Autodesk Inventor part; units mm, degrees
(part 4 of 5)
  line L871 (-97.2926, -57.6618) -> (-97.2926, -57.0118) projected
  line L872 (-97.2926, -49.1118) -> (-95.6926, -49.1118) projected
  line L873 (-95.6926, -49.1118) -> (-95.6926, -49.7618) projected
  line L874 (-95.6926, -49.7618) -> (-97.2926, -49.7618) projected
  line L875 (-97.2926, -49.7618) -> (-97.2926, -49.1118) projected
  line L876 (-98.1576, -55.9868) -> (-97.3676, -55.9868) projected
  line L877 (-97.3676, -55.9868) -> (-97.3676, -56.3868) projected
  line L878 (-97.3676, -56.3868) -> (-98.1576, -56.3868) projected
  line L879 (-98.1576, -56.3868) -> (-98.1576, -55.9868) projected
  line L880 (-95.6176, -55.9868) -> (-94.8276, -55.9868) projected
  line L881 (-94.8276, -55.9868) -> (-94.8276, -56.3868) projected
  line L882 (-94.8276, -56.3868) -> (-95.6176, -56.3868) projected
  line L883 (-95.6176, -56.3868) -> (-95.6176, -55.9868) projected
  line L884 (-98.1576, -55.1868) -> (-97.3676, -55.1868) projected
  line L885 (-97.3676, -55.1868) -> (-97.3676, -55.5868) projected
  line L886 (-97.3676, -55.5868) -> (-98.1576, -55.5868) projected
  line L887 (-98.1576, -55.5868) -> (-98.1576, -55.1868) projected
  line L888 (-95.6176, -55.1868) -> (-94.8276, -55.1868) projected
  line L889 (-94.8276, -55.1868) -> (-94.8276, -55.5868) projected
  line L890 (-94.8276, -55.5868) -> (-95.6176, -55.5868) projected
  line L891 (-95.6176, -55.5868) -> (-95.6176, -55.1868) projected
  line L892 (-98.1576, -54.3868) -> (-97.3676, -54.3868) projected
  line L893 (-97.3676, -54.3868) -> (-97.3676, -54.7868) projected
  line L894 (-97.3676, -54.7868) -> (-98.1576, -54.7868) projected
  line L895 (-98.1576, -54.7868) -> (-98.1576, -54.3868) projected
  line L896 (-95.6176, -54.3868) -> (-94.8276, -54.3868) projected
  line L897 (-94.8276, -54.3868) -> (-94.8276, -54.7868) projected
  line L898 (-94.8276, -54.7868) -> (-95.6176, -54.7868) projected
  line L899 (-95.6176, -54.7868) -> (-95.6176, -54.3868) projected
  line L900 (-98.1576, -53.5868) -> (-97.3676, -53.5868) projected
  line L901 (-97.3676, -53.5868) -> (-97.3676, -53.9868) projected
  line L902 (-97.3676, -53.9868) -> (-98.1576, -53.9868) projected
  line L903 (-98.1576, -53.9868) -> (-98.1576, -53.5868) projected
  line L904 (-95.6176, -53.5868) -> (-94.8276, -53.5868) projected
  line L905 (-94.8276, -53.5868) -> (-94.8276, -53.9868) projected
  line L906 (-94.8276, -53.9868) -> (-95.6176, -53.9868) projected
  line L907 (-95.6176, -53.9868) -> (-95.6176, -53.5868) projected
  line L908 (-98.1576, -52.7868) -> (-97.3676, -52.7868) projected
  line L909 (-97.3676, -52.7868) -> (-97.3676, -53.1868) projected
  line L910 (-97.3676, -53.1868) -> (-98.1576, -53.1868) projected
  line L911 (-98.1576, -53.1868) -> (-98.1576, -52.7868) projected
  line L912 (-95.6176, -52.7868) -> (-94.8276, -52.7868) projected
  line L913 (-94.8276, -52.7868) -> (-94.8276, -53.1868) projected
  line L914 (-94.8276, -53.1868) -> (-95.6176, -53.1868) projected
  line L915 (-95.6176, -53.1868) -> (-95.6176, -52.7868) projected
  line L916 (-98.1576, -51.9868) -> (-97.3676, -51.9868) projected
  line L917 (-97.3676, -51.9868) -> (-97.3676, -52.3868) projected
  line L918 (-97.3676, -52.3868) -> (-98.1576, -52.3868) projected
  line L919 (-98.1576, -52.3868) -> (-98.1576, -51.9868) projected
  line L920 (-95.6176, -51.9868) -> (-94.8276, -51.9868) projected
  line L921 (-94.8276, -51.9868) -> (-94.8276, -52.3868) projected
  line L922 (-94.8276, -52.3868) -> (-95.6176, -52.3868) projected
  line L923 (-95.6176, -52.3868) -> (-95.6176, -51.9868) projected
  line L924 (-98.1576, -51.1868) -> (-97.3676, -51.1868) projected
  line L925 (-97.3676, -51.1868) -> (-97.3676, -51.5868) projected
  line L926 (-97.3676, -51.5868) -> (-98.1576, -51.5868) projected
  line L927 (-98.1576, -51.5868) -> (-98.1576, -51.1868) projected
  line L928 (-95.6176, -51.1868) -> (-94.8276, -51.1868) projected
  line L929 (-94.8276, -51.1868) -> (-94.8276, -51.5868) projected
  line L930 (-94.8276, -51.5868) -> (-95.6176, -51.5868) projected
  line L931 (-95.6176, -51.5868) -> (-95.6176, -51.1868) projected
  line L932 (-98.1576, -50.3868) -> (-97.3676, -50.3868) projected
  line L933 (-97.3676, -50.3868) -> (-97.3676, -50.7868) projected
  line L934 (-97.3676, -50.7868) -> (-98.1576, -50.7868) projected
  line L935 (-98.1576, -50.7868) -> (-98.1576, -50.3868) projected
  line L936 (-95.6176, -50.3868) -> (-94.8276, -50.3868) projected
  line L937 (-94.8276, -50.3868) -> (-94.8276, -50.7868) projected
  line L938 (-94.8276, -50.7868) -> (-95.6176, -50.7868) projected
  line L939 (-95.6176, -50.7868) -> (-95.6176, -50.3868) projected
  line L940 (-59.7501, -19.4368) -> (-58.1501, -19.4368) projected
  line L941 (-58.1501, -19.4368) -> (-58.1501, -20.0868) projected
  line L942 (-58.1501, -20.0868) -> (-59.7501, -20.0868) projected
  line L943 (-59.7501, -20.0868) -> (-59.7501, -19.4368) projected
  line L944 (-59.7501, -11.5368) -> (-58.1501, -11.5368) projected
  line L945 (-58.1501, -11.5368) -> (-58.1501, -12.1868) projected
  line L946 (-58.1501, -12.1868) -> (-59.7501, -12.1868) projected
  line L947 (-59.7501, -12.1868) -> (-59.7501, -11.5368) projected
  line L948 (-60.6151, -18.4118) -> (-59.8251, -18.4118) projected
  line L949 (-59.8251, -18.4118) -> (-59.8251, -18.8118) projected
  line L950 (-59.8251, -18.8118) -> (-60.6151, -18.8118) projected
  line L951 (-60.6151, -18.8118) -> (-60.6151, -18.4118) projected
  line L952 (-58.0751, -18.4118) -> (-57.2851, -18.4118) projected
  line L953 (-57.2851, -18.4118) -> (-57.2851, -18.8118) projected
  line L954 (-57.2851, -18.8118) -> (-58.0751, -18.8118) projected
  line L955 (-58.0751, -18.8118) -> (-58.0751, -18.4118) projected
  line L956 (-60.6151, -17.6118) -> (-59.8251, -17.6118) projected
  line L957 (-59.8251, -17.6118) -> (-59.8251, -18.0118) projected
  line L958 (-59.8251, -18.0118) -> (-60.6151, -18.0118) projected
  line L959 (-60.6151, -18.0118) -> (-60.6151, -17.6118) projected
  line L960 (-58.0751, -17.6118) -> (-57.2851, -17.6118) projected
  line L961 (-57.2851, -17.6118) -> (-57.2851, -18.0118) projected
  line L962 (-57.2851, -18.0118) -> (-58.0751, -18.0118) projected
  line L963 (-58.0751, -18.0118) -> (-58.0751, -17.6118) projected
  line L964 (-60.6151, -16.8118) -> (-59.8251, -16.8118) projected
  line L965 (-59.8251, -16.8118) -> (-59.8251, -17.2118) projected
  line L966 (-59.8251, -17.2118) -> (-60.6151, -17.2118) projected
  line L967 (-60.6151, -17.2118) -> (-60.6151, -16.8118) projected
  line L968 (-58.0751, -16.8118) -> (-57.2851, -16.8118) projected
  line L969 (-57.2851, -16.8118) -> (-57.2851, -17.2118) projected
  line L970 (-57.2851, -17.2118) -> (-58.0751, -17.2118) projected
  line L971 (-58.0751, -17.2118) -> (-58.0751, -16.8118) projected
  line L972 (-60.6151, -16.0118) -> (-59.8251, -16.0118) projected
  line L973 (-59.8251, -16.0118) -> (-59.8251, -16.4118) projected
  line L974 (-59.8251, -16.4118) -> (-60.6151, -16.4118) projected
  line L975 (-60.6151, -16.4118) -> (-60.6151, -16.0118) projected
  line L976 (-58.0751, -16.0118) -> (-57.2851, -16.0118) projected
  line L977 (-57.2851, -16.0118) -> (-57.2851, -16.4118) projected
  line L978 (-57.2851, -16.4118) -> (-58.0751, -16.4118) projected
  line L979 (-58.0751, -16.4118) -> (-58.0751, -16.0118) projected
  line L980 (-60.6151, -15.2118) -> (-59.8251, -15.2118) projected
  line L981 (-59.8251, -15.2118) -> (-59.8251, -15.6118) projected
  line L982 (-59.8251, -15.6118) -> (-60.6151, -15.6118) projected
  line L983 (-60.6151, -15.6118) -> (-60.6151, -15.2118) projected
  line L984 (-58.0751, -15.2118) -> (-57.2851, -15.2118) projected
  line L985 (-57.2851, -15.2118) -> (-57.2851, -15.6118) projected
  line L986 (-57.2851, -15.6118) -> (-58.0751, -15.6118) projected
  line L987 (-58.0751, -15.6118) -> (-58.0751, -15.2118) projected
  line L988 (-60.6151, -14.4118) -> (-59.8251, -14.4118) projected
  line L989 (-59.8251, -14.4118) -> (-59.8251, -14.8118) projected
  line L990 (-59.8251, -14.8118) -> (-60.6151, -14.8118) projected
  line L991 (-60.6151, -14.8118) -> (-60.6151, -14.4118) projected
  line L992 (-58.0751, -14.4118) -> (-57.2851, -14.4118) projected
  line L993 (-57.2851, -14.4118) -> (-57.2851, -14.8118) projected
  line L994 (-57.2851, -14.8118) -> (-58.0751, -14.8118) projected
  line L995 (-58.0751, -14.8118) -> (-58.0751, -14.4118) projected
  line L996 (-60.6151, -13.6118) -> (-59.8251, -13.6118) projected
  line L997 (-59.8251, -13.6118) -> (-59.8251, -14.0118) projected
  line L998 (-59.8251, -14.0118) -> (-60.6151, -14.0118) projected
  line L999 (-60.6151, -14.0118) -> (-60.6151, -13.6118) projected
  line L1000 (-58.0751, -13.6118) -> (-57.2851, -13.6118) projected
  line L1001 (-57.2851, -13.6118) -> (-57.2851, -14.0118) projected
  line L1002 (-57.2851, -14.0118) -> (-58.0751, -14.0118) projected
  line L1003 (-58.0751, -14.0118) -> (-58.0751, -13.6118) projected
  line L1004 (-60.6151, -12.8118) -> (-59.8251, -12.8118) projected
  line L1005 (-59.8251, -12.8118) -> (-59.8251, -13.2118) projected
  line L1006 (-59.8251, -13.2118) -> (-60.6151, -13.2118) projected
  line L1007 (-60.6151, -13.2118) -> (-60.6151, -12.8118) projected
  line L1008 (-58.0751, -12.8118) -> (-57.2851, -12.8118) projected
  line L1009 (-57.2851, -12.8118) -> (-57.2851, -13.2118) projected
  line L1010 (-57.2851, -13.2118) -> (-58.0751, -13.2118) projected
  line L1011 (-58.0751, -13.2118) -> (-58.0751, -12.8118) projected
  line L1012 (-116.5001, -19.3118) -> (-114.9001, -19.3118) projected
  line L1013 (-114.9001, -19.3118) -> (-114.9001, -19.9618) projected
  line L1014 (-114.9001, -19.9618) -> (-116.5001, -19.9618) projected
  line L1015 (-116.5001, -19.9618) -> (-116.5001, -19.3118) projected
  line L1016 (-116.5001, -11.4118) -> (-114.9001, -11.4118) projected
  line L1017 (-114.9001, -11.4118) -> (-114.9001, -12.0618) projected
  line L1018 (-114.9001, -12.0618) -> (-116.5001, -12.0618) projected
  line L1019 (-116.5001, -12.0618) -> (-116.5001, -11.4118) projected
  line L1020 (-117.3651, -18.2868) -> (-116.5751, -18.2868) projected
  line L1021 (-116.5751, -18.2868) -> (-116.5751, -18.6868) projected
  line L1022 (-116.5751, -18.6868) -> (-117.3651, -18.6868) projected
  line L1023 (-117.3651, -18.6868) -> (-117.3651, -18.2868) projected
  line L1024 (-114.8251, -18.2868) -> (-114.0351, -18.2868) projected
  line L1025 (-114.0351, -18.2868) -> (-114.0351, -18.6868) projected
  line L1026 (-114.0351, -18.6868) -> (-114.8251, -18.6868) projected
  line L1027 (-114.8251, -18.6868) -> (-114.8251, -18.2868) projected
  line L1028 (-117.3651, -17.4868) -> (-116.5751, -17.4868) projected
  line L1029 (-116.5751, -17.4868) -> (-116.5751, -17.8868) projected
  line L1030 (-116.5751, -17.8868) -> (-117.3651, -17.8868) projected
  line L1031 (-117.3651, -17.8868) -> (-117.3651, -17.4868) projected
  line L1032 (-114.8251, -17.4868) -> (-114.0351, -17.4868) projected
  line L1033 (-114.0351, -17.4868) -> (-114.0351, -17.8868) projected
  line L1034 (-114.0351, -17.8868) -> (-114.8251, -17.8868) projected
  line L1035 (-114.8251, -17.8868) -> (-114.8251, -17.4868) projected
  line L1036 (-117.3651, -16.6868) -> (-116.5751, -16.6868) projected
  line L1037 (-116.5751, -16.6868) -> (-116.5751, -17.0868) projected
  line L1038 (-116.5751, -17.0868) -> (-117.3651, -17.0868) projected
  line L1039 (-117.3651, -17.0868) -> (-117.3651, -16.6868) projected
  line L1040 (-114.8251, -16.6868) -> (-114.0351, -16.6868) projected
  line L1041 (-114.0351, -16.6868) -> (-114.0351, -17.0868) projected
  line L1042 (-114.0351, -17.0868) -> (-114.8251, -17.0868) projected
  line L1043 (-114.8251, -17.0868) -> (-114.8251, -16.6868) projected
  line L1044 (-117.3651, -15.8868) -> (-116.5751, -15.8868) projected
  line L1045 (-116.5751, -15.8868) -> (-116.5751, -16.2868) projected
  line L1046 (-116.5751, -16.2868) -> (-117.3651, -16.2868) projected
  line L1047 (-117.3651, -16.2868) -> (-117.3651, -15.8868) projected
  line L1048 (-114.8251, -15.8868) -> (-114.0351, -15.8868) projected
  line L1049 (-114.0351, -15.8868) -> (-114.0351, -16.2868) projected
  line L1050 (-114.0351, -16.2868) -> (-114.8251, -16.2868) projected
  line L1051 (-114.8251, -16.2868) -> (-114.8251, -15.8868) projected
  line L1052 (-117.3651, -15.0868) -> (-116.5751, -15.0868) projected
  line L1053 (-116.5751, -15.0868) -> (-116.5751, -15.4868) projected
  line L1054 (-116.5751, -15.4868) -> (-117.3651, -15.4868) projected
  line L1055 (-117.3651, -15.4868) -> (-117.3651, -15.0868) projected
  line L1056 (-114.8251, -15.0868) -> (-114.0351, -15.0868) projected
  line L1057 (-114.0351, -15.0868) -> (-114.0351, -15.4868) projected
  line L1058 (-114.0351, -15.4868) -> (-114.8251, -15.4868) projected
  line L1059 (-114.8251, -15.4868) -> (-114.8251, -15.0868) projected
  line L1060 (-117.3651, -14.2868) -> (-116.5751, -14.2868) projected
  line L1061 (-116.5751, -14.2868) -> (-116.5751, -14.6868) projected
  line L1062 (-116.5751, -14.6868) -> (-117.3651, -14.6868) projected
  line L1063 (-117.3651, -14.6868) -> (-117.3651, -14.2868) projected
  line L1064 (-114.8251, -14.2868) -> (-114.0351, -14.2868) projected
  line L1065 (-114.0351, -14.2868) -> (-114.0351, -14.6868) projected
  line L1066 (-114.0351, -14.6868) -> (-114.8251, -14.6868) projected
  line L1067 (-114.8251, -14.6868) -> (-114.8251, -14.2868) projected
  line L1068 (-117.3651, -13.4868) -> (-116.5751, -13.4868) projected
  line L1069 (-116.5751, -13.4868) -> (-116.5751, -13.8868) projected
  line L1070 (-116.5751, -13.8868) -> (-117.3651, -13.8868) projected
  line L1071 (-117.3651, -13.8868) -> (-117.3651, -13.4868) projected
  line L1072 (-114.8251, -13.4868) -> (-114.0351, -13.4868) projected
  line L1073 (-114.0351, -13.4868) -> (-114.0351, -13.8868) projected
  line L1074 (-114.0351, -13.8868) -> (-114.8251, -13.8868) projected
  line L1075 (-114.8251, -13.8868) -> (-114.8251, -13.4868) projected
  line L1076 (-117.3651, -12.6868) -> (-116.5751, -12.6868) projected
  line L1077 (-116.5751, -12.6868) -> (-116.5751, -13.0868) projected
  line L1078 (-116.5751, -13.0868) -> (-117.3651, -13.0868) projected
  line L1079 (-117.3651, -13.0868) -> (-117.3651, -12.6868) projected
  line L1080 (-114.8251, -12.6868) -> (-114.0351, -12.6868) projected
  line L1081 (-114.0351, -12.6868) -> (-114.0351, -13.0868) projected
  line L1082 (-114.0351, -13.0868) -> (-114.8251, -13.0868) projected
  line L1083 (-114.8251, -13.0868) -> (-114.8251, -12.6868) projected
  line L1084 (-40.9426, -19.3618) -> (-39.3426, -19.3618) projected
  line L1085 (-39.3426, -19.3618) -> (-39.3426, -20.0118) projected
  line L1086 (-39.3426, -20.0118) -> (-40.9426, -20.0118) projected
  line L1087 (-40.9426, -20.0118) -> (-40.9426, -19.3618) projected
  line L1088 (-40.9426, -11.4618) -> (-39.3426, -11.4618) projected
  line L1089 (-39.3426, -11.4618) -> (-39.3426, -12.1118) projected
  line L1090 (-39.3426, -12.1118) -> (-40.9426, -12.1118) projected
  line L1091 (-40.9426, -12.1118) -> (-40.9426, -11.4618) projected
  line L1092 (-41.8076, -18.3368) -> (-41.0176, -18.3368) projected
  line L1093 (-41.0176, -18.3368) -> (-41.0176, -18.7368) projected
  line L1094 (-41.0176, -18.7368) -> (-41.8076, -18.7368) projected
  line L1095 (-41.8076, -18.7368) -> (-41.8076, -18.3368) projected
  line L1096 (-39.2676, -18.3368) -> (-38.4776, -18.3368) projected
  line L1097 (-38.4776, -18.3368) -> (-38.4776, -18.7368) projected
  line L1098 (-38.4776, -18.7368) -> (-39.2676, -18.7368) projected
  line L1099 (-39.2676, -18.7368) -> (-39.2676, -18.3368) projected
  line L1100 (-41.8076, -17.5368) -> (-41.0176, -17.5368) projected
  line L1101 (-41.0176, -17.5368) -> (-41.0176, -17.9368) projected
  line L1102 (-41.0176, -17.9368) -> (-41.8076, -17.9368) projected
  line L1103 (-41.8076, -17.9368) -> (-41.8076, -17.5368) projected
  line L1104 (-39.2676, -17.5368) -> (-38.4776, -17.5368) projected
  line L1105 (-38.4776, -17.5368) -> (-38.4776, -17.9368) projected
  line L1106 (-38.4776, -17.9368) -> (-39.2676, -17.9368) projected
  line L1107 (-39.2676, -17.9368) -> (-39.2676, -17.5368) projected
  line L1108 (-41.8076, -16.7368) -> (-41.0176, -16.7368) projected
  line L1109 (-41.0176, -16.7368) -> (-41.0176, -17.1368) projected
  line L1110 (-41.0176, -17.1368) -> (-41.8076, -17.1368) projected
  line L1111 (-41.8076, -17.1368) -> (-41.8076, -16.7368) projected
  line L1112 (-39.2676, -16.7368) -> (-38.4776, -16.7368) projected
  line L1113 (-38.4776, -16.7368) -> (-38.4776, -17.1368) projected
  line L1114 (-38.4776, -17.1368) -> (-39.2676, -17.1368) projected
  line L1115 (-39.2676, -17.1368) -> (-39.2676, -16.7368) projected
  line L1116 (-41.8076, -15.9368) -> (-41.0176, -15.9368) projected
  line L1117 (-41.0176, -15.9368) -> (-41.0176, -16.3368) projected
  line L1118 (-41.0176, -16.3368) -> (-41.8076, -16.3368) projected
  line L1119 (-41.8076, -16.3368) -> (-41.8076, -15.9368) projected
  line L1120 (-39.2676, -15.9368) -> (-38.4776, -15.9368) projected
  line L1121 (-38.4776, -15.9368) -> (-38.4776, -16.3368) projected
  line L1122 (-38.4776, -16.3368) -> (-39.2676, -16.3368) projected
  line L1123 (-39.2676, -16.3368) -> (-39.2676, -15.9368) projected
  line L1124 (-41.8076, -15.1368) -> (-41.0176, -15.1368) projected
  line L1125 (-41.0176, -15.1368) -> (-41.0176, -15.5368) projected
  line L1126 (-41.0176, -15.5368) -> (-41.8076, -15.5368) projected
  line L1127 (-41.8076, -15.5368) -> (-41.8076, -15.1368) projected
  line L1128 (-39.2676, -15.1368) -> (-38.4776, -15.1368) projected
  line L1129 (-38.4776, -15.1368) -> (-38.4776, -15.5368) projected
  line L1130 (-38.4776, -15.5368) -> (-39.2676, -15.5368) projected
  line L1131 (-39.2676, -15.5368) -> (-39.2676, -15.1368) projected
  line L1132 (-41.8076, -14.3368) -> (-41.0176, -14.3368) projected
  line L1133 (-41.0176, -14.3368) -> (-41.0176, -14.7368) projected
  line L1134 (-41.0176, -14.7368) -> (-41.8076, -14.7368) projected
  line L1135 (-41.8076, -14.7368) -> (-41.8076, -14.3368) projected
  line L1136 (-39.2676, -14.3368) -> (-38.4776, -14.3368) projected
  line L1137 (-38.4776, -14.3368) -> (-38.4776, -14.7368) projected
  line L1138 (-38.4776, -14.7368) -> (-39.2676, -14.7368) projected
  line L1139 (-39.2676, -14.7368) -> (-39.2676, -14.3368) projected
  line L1140 (-41.8076, -13.5368) -> (-41.0176, -13.5368) projected
  line L1141 (-41.0176, -13.5368) -> (-41.0176, -13.9368) projected
  line L1142 (-41.0176, -13.9368) -> (-41.8076, -13.9368) projected
  line L1143 (-41.8076, -13.9368) -> (-41.8076, -13.5368) projected
  line L1144 (-39.2676, -13.5368) -> (-38.4776, -13.5368) projected
  line L1145 (-38.4776, -13.5368) -> (-38.4776, -13.9368) projected
  line L1146 (-38.4776, -13.9368) -> (-39.2676, -13.9368) projected
  line L1147 (-39.2676, -13.9368) -> (-39.2676, -13.5368) projected
  line L1148 (-41.8076, -12.7368) -> (-41.0176, -12.7368) projected
  line L1149 (-41.0176, -12.7368) -> (-41.0176, -13.1368) projected
  line L1150 (-41.0176, -13.1368) -> (-41.8076, -13.1368) projected
  line L1151 (-41.8076, -13.1368) -> (-41.8076, -12.7368) projected
  line L1152 (-39.2676, -12.7368) -> (-38.4776, -12.7368) projected
  line L1153 (-38.4776, -12.7368) -> (-38.4776, -13.1368) projected
  line L1154 (-38.4776, -13.1368) -> (-39.2676, -13.1368) projected
  line L1155 (-39.2676, -13.1368) -> (-39.2676, -12.7368) projected
  line L1156 (-40.7851, -57.0368) -> (-39.1851, -57.0368) projected
  line L1157 (-39.1851, -57.0368) -> (-39.1851, -57.6868) projected
  line L1158 (-39.1851, -57.6868) -> (-40.7851, -57.6868) projected
  line L1159 (-40.7851, -57.6868) -> (-40.7851, -57.0368) projected
  line L1160 (-40.7851, -49.1368) -> (-39.1851, -49.1368) projected
  line L1161 (-39.1851, -49.1368) -> (-39.1851, -49.7868) projected
  line L1162 (-39.1851, -49.7868) -> (-40.7851, -49.7868) projected
  line L1163 (-40.7851, -49.7868) -> (-40.7851, -49.1368) projected
  line L1164 (-41.6501, -56.0118) -> (-40.8601, -56.0118) projected
  line L1165 (-40.8601, -56.0118) -> (-40.8601, -56.4118) projected
  line L1166 (-40.8601, -56.4118) -> (-41.6501, -56.4118) projected
  line L1167 (-41.6501, -56.4118) -> (-41.6501, -56.0118) projected
  line L1168 (-39.1101, -56.0118) -> (-38.3201, -56.0118) projected
  line L1169 (-38.3201, -56.0118) -> (-38.3201, -56.4118) projected
  line L1170 (-38.3201, -56.4118) -> (-39.1101, -56.4118) projected
  line L1171 (-39.1101, -56.4118) -> (-39.1101, -56.0118) projected
  line L1172 (-41.6501, -55.2118) -> (-40.8601, -55.2118) projected
  line L1173 (-40.8601, -55.2118) -> (-40.8601, -55.6118) projected
  line L1174 (-40.8601, -55.6118) -> (-41.6501, -55.6118) projected
  line L1175 (-41.6501, -55.6118) -> (-41.6501, -55.2118) projected
  line L1176 (-39.1101, -55.2118) -> (-38.3201, -55.2118) projected
  line L1177 (-38.3201, -55.2118) -> (-38.3201, -55.6118) projected
  line L1178 (-38.3201, -55.6118) -> (-39.1101, -55.6118) projected
  line L1179 (-39.1101, -55.6118) -> (-39.1101, -55.2118) projected
  line L1180 (-41.6501, -54.4118) -> (-40.8601, -54.4118) projected
  line L1181 (-40.8601, -54.4118) -> (-40.8601, -54.8118) projected
  line L1182 (-40.8601, -54.8118) -> (-41.6501, -54.8118) projected
  line L1183 (-41.6501, -54.8118) -> (-41.6501, -54.4118) projected
  line L1184 (-39.1101, -54.4118) -> (-38.3201, -54.4118) projected
  line L1185 (-38.3201, -54.4118) -> (-38.3201, -54.8118) projected
  line L1186 (-38.3201, -54.8118) -> (-39.1101, -54.8118) projected
  line L1187 (-39.1101, -54.8118) -> (-39.1101, -54.4118) projected
  line L1188 (-41.6501, -53.6118) -> (-40.8601, -53.6118) projected
  line L1189 (-40.8601, -53.6118) -> (-40.8601, -54.0118) projected
  line L1190 (-40.8601, -54.0118) -> (-41.6501, -54.0118) projected
  line L1191 (-41.6501, -54.0118) -> (-41.6501, -53.6118) projected
  line L1192 (-39.1101, -53.6118) -> (-38.3201, -53.6118) projected
  line L1193 (-38.3201, -53.6118) -> (-38.3201, -54.0118) projected
  line L1194 (-38.3201, -54.0118) -> (-39.1101, -54.0118) projected
  line L1195 (-39.1101, -54.0118) -> (-39.1101, -53.6118) projected
  line L1196 (-41.6501, -52.8118) -> (-40.8601, -52.8118) projected
  line L1197 (-40.8601, -52.8118) -> (-40.8601, -53.2118) projected
  line L1198 (-40.8601, -53.2118) -> (-41.6501, -53.2118) projected
  line L1199 (-41.6501, -53.2118) -> (-41.6501, -52.8118) projected
  line L1200 (-39.1101, -52.8118) -> (-38.3201, -52.8118) projected
  line L1201 (-38.3201, -52.8118) -> (-38.3201, -53.2118) projected
  line L1202 (-38.3201, -53.2118) -> (-39.1101, -53.2118) projected
  line L1203 (-39.1101, -53.2118) -> (-39.1101, -52.8118) projected
  line L1204 (-41.6501, -52.0118) -> (-40.8601, -52.0118) projected
  line L1205 (-40.8601, -52.0118) -> (-40.8601, -52.4118) projected
  line L1206 (-40.8601, -52.4118) -> (-41.6501, -52.4118) projected
  line L1207 (-41.6501, -52.4118) -> (-41.6501, -52.0118) projected
  line L1208 (-39.1101, -52.0118) -> (-38.3201, -52.0118) projected
  line L1209 (-38.3201, -52.0118) -> (-38.3201, -52.4118) projected
  line L1210 (-38.3201, -52.4118) -> (-39.1101, -52.4118) projected
  line L1211 (-39.1101, -52.4118) -> (-39.1101, -52.0118) projected
  line L1212 (-41.6501, -51.2118) -> (-40.8601, -51.2118) projected
  line L1213 (-40.8601, -51.2118) -> (-40.8601, -51.6118) projected
  line L1214 (-40.8601, -51.6118) -> (-41.6501, -51.6118) projected
  line L1215 (-41.6501, -51.6118) -> (-41.6501, -51.2118) projected
  line L1216 (-39.1101, -51.2118) -> (-38.3201, -51.2118) projected
  line L1217 (-38.3201, -51.2118) -> (-38.3201, -51.6118) projected
  line L1218 (-38.3201, -51.6118) -> (-39.1101, -51.6118) projected
  line L1219 (-39.1101, -51.6118) -> (-39.1101, -51.2118) projected
  line L1220 (-41.6501, -50.4118) -> (-40.8601, -50.4118) projected
  line L1221 (-40.8601, -50.4118) -> (-40.8601, -50.8118) projected
  line L1222 (-40.8601, -50.8118) -> (-41.6501, -50.8118) projected
  line L1223 (-41.6501, -50.8118) -> (-41.6501, -50.4118) projected
  line L1224 (-39.1101, -50.4118) -> (-38.3201, -50.4118) projected
  line L1225 (-38.3201, -50.4118) -> (-38.3201, -50.8118) projected
  line L1226 (-38.3201, -50.8118) -> (-39.1101, -50.8118) projected
  line L1227 (-39.1101, -50.8118) -> (-39.1101, -50.4118) projected
  line L1228 (-78.4676, -57.1118) -> (-76.8676, -57.1118) projected
  line L1229 (-76.8676, -57.1118) -> (-76.8676, -57.7618) projected
  line L1230 (-76.8676, -57.7618) -> (-78.4676, -57.7618) projected
  line L1231 (-78.4676, -57.7618) -> (-78.4676, -57.1118) projected
  line L1232 (-78.4676, -49.2118) -> (-76.8676, -49.2118) projected
  line L1233 (-76.8676, -49.2118) -> (-76.8676, -49.8618) projected
  line L1234 (-76.8676, -49.8618) -> (-78.4676, -49.8618) projected
  line L1235 (-78.4676, -49.8618) -> (-78.4676, -49.2118) projected
  line L1236 (-79.3326, -56.0868) -> (-78.5426, -56.0868) projected
  line L1237 (-78.5426, -56.0868) -> (-78.5426, -56.4868) projected
  line L1238 (-78.5426, -56.4868) -> (-79.3326, -56.4868) projected
  line L1239 (-79.3326, -56.4868) -> (-79.3326, -56.0868) projected
  line L1240 (-76.7926, -56.0868) -> (-76.0026, -56.0868) projected
  line L1241 (-76.0026, -56.0868) -> (-76.0026, -56.4868) projected
  line L1242 (-76.0026, -56.4868) -> (-76.7926, -56.4868) projected
  line L1243 (-76.7926, -56.4868) -> (-76.7926, -56.0868) projected
  line L1244 (-79.3326, -55.2868) -> (-78.5426, -55.2868) projected
  line L1245 (-78.5426, -55.2868) -> (-78.5426, -55.6868) projected
  line L1246 (-78.5426, -55.6868) -> (-79.3326, -55.6868) projected
  line L1247 (-79.3326, -55.6868) -> (-79.3326, -55.2868) projected
  line L1248 (-76.7926, -55.2868) -> (-76.0026, -55.2868) projected
  line L1249 (-76.0026, -55.2868) -> (-76.0026, -55.6868) projected
  line L1250 (-76.0026, -55.6868) -> (-76.7926, -55.6868) projected
  line L1251 (-76.7926, -55.6868) -> (-76.7926, -55.2868) projected
  line L1252 (-79.3326, -54.4868) -> (-78.5426, -54.4868) projected
  line L1253 (-78.5426, -54.4868) -> (-78.5426, -54.8868) projected
  line L1254 (-78.5426, -54.8868) -> (-79.3326, -54.8868) projected
  line L1255 (-79.3326, -54.8868) -> (-79.3326, -54.4868) projected
  line L1256 (-76.7926, -54.4868) -> (-76.0026, -54.4868) projected
  line L1257 (-76.0026, -54.4868) -> (-76.0026, -54.8868) projected
  line L1258 (-76.0026, -54.8868) -> (-76.7926, -54.8868) projected
  line L1259 (-76.7926, -54.8868) -> (-76.7926, -54.4868) projected
  line L1260 (-79.3326, -53.6868) -> (-78.5426, -53.6868) projected
  line L1261 (-78.5426, -53.6868) -> (-78.5426, -54.0868) projected
  line L1262 (-78.5426, -54.0868) -> (-79.3326, -54.0868) projected
  line L1263 (-79.3326, -54.0868) -> (-79.3326, -53.6868) projected
  line L1264 (-76.7926, -53.6868) -> (-76.0026, -53.6868) projected
  line L1265 (-76.0026, -53.6868) -> (-76.0026, -54.0868) projected
  line L1266 (-76.0026, -54.0868) -> (-76.7926, -54.0868) projected
  line L1267 (-76.7926, -54.0868) -> (-76.7926, -53.6868) projected
  line L1268 (-79.3326, -52.8868) -> (-78.5426, -52.8868) projected
  line L1269 (-78.5426, -52.8868) -> (-78.5426, -53.2868) projected
  line L1270 (-78.5426, -53.2868) -> (-79.3326, -53.2868) projected
  line L1271 (-79.3326, -53.2868) -> (-79.3326, -52.8868) projected
  line L1272 (-76.7926, -52.8868) -> (-76.0026, -52.8868) projected
  line L1273 (-76.0026, -52.8868) -> (-76.0026, -53.2868) projected
  line L1274 (-76.0026, -53.2868) -> (-76.7926, -53.2868) projected
  line L1275 (-76.7926, -53.2868) -> (-76.7926, -52.8868) projected
  line L1276 (-79.3326, -52.0868) -> (-78.5426, -52.0868) projected
  line L1277 (-78.5426, -52.0868) -> (-78.5426, -52.4868) projected
  line L1278 (-78.5426, -52.4868) -> (-79.3326, -52.4868) projected
  line L1279 (-79.3326, -52.4868) -> (-79.3326, -52.0868) projected
  line L1280 (-76.7926, -52.0868) -> (-76.0026, -52.0868) projected
  line L1281 (-76.0026, -52.0868) -> (-76.0026, -52.4868) projected
  line L1282 (-76.0026, -52.4868) -> (-76.7926, -52.4868) projected
  line L1283 (-76.7926, -52.4868) -> (-76.7926, -52.0868) projected
  line L1284 (-79.3326, -51.2868) -> (-78.5426, -51.2868) projected
  line L1285 (-78.5426, -51.2868) -> (-78.5426, -51.6868) projected
  line L1286 (-78.5426, -51.6868) -> (-79.3326, -51.6868) projected
  line L1287 (-79.3326, -51.6868) -> (-79.3326, -51.2868) projected
  line L1288 (-76.7926, -51.2868) -> (-76.0026, -51.2868) projected
  line L1289 (-76.0026, -51.2868) -> (-76.0026, -51.6868) projected
  line L1290 (-76.0026, -51.6868) -> (-76.7926, -51.6868) projected
  line L1291 (-76.7926, -51.6868) -> (-76.7926, -51.2868) projected
  line L1292 (-79.3326, -50.4868) -> (-78.5426, -50.4868) projected
  line L1293 (-78.5426, -50.4868) -> (-78.5426, -50.8868) projected
  line L1294 (-78.5426, -50.8868) -> (-79.3326, -50.8868) projected
  line L1295 (-79.3326, -50.8868) -> (-79.3326, -50.4868) projected
  line L1296 (-76.7926, -50.4868) -> (-76.0026, -50.4868) projected
  line L1297 (-76.0026, -50.4868) -> (-76.0026, -50.8868) projected
  line L1298 (-76.0026, -50.8868) -> (-76.7926, -50.8868) projected
  line L1299 (-76.7926, -50.8868) -> (-76.7926, -50.4868) projected
  line L1300 (-58.2076, -68.4118) -> (-59.8076, -68.4118) projected
  line L1301 (-59.8076, -68.4118) -> (-59.8076, -67.7618) projected
  line L1302 (-59.8076, -67.7618) -> (-58.2076, -67.7618) projected
  line L1303 (-58.2076, -67.7618) -> (-58.2076, -68.4118) projected
  line L1304 (-58.2076, -76.3118) -> (-59.8076, -76.3118) projected
  line L1305 (-59.8076, -76.3118) -> (-59.8076, -75.6618) projected
  line L1306 (-59.8076, -75.6618) -> (-58.2076, -75.6618) projected
  line L1307 (-58.2076, -75.6618) -> (-58.2076, -76.3118) projected
  line L1308 (-57.3426, -69.4368) -> (-58.1326, -69.4368) projected
  line L1309 (-58.1326, -69.4368) -> (-58.1326, -69.0368) projected
  line L1310 (-58.1326, -69.0368) -> (-57.3426, -69.0368) projected
  line L1311 (-57.3426, -69.0368) -> (-57.3426, -69.4368) projected
  line L1312 (-59.8826, -69.4368) -> (-60.6726, -69.4368) projected
  line L1313 (-60.6726, -69.4368) -> (-60.6726, -69.0368) projected
  line L1314 (-60.6726, -69.0368) -> (-59.8826, -69.0368) projected
  line L1315 (-59.8826, -69.0368) -> (-59.8826, -69.4368) projected
  line L1316 (-57.3426, -70.2368) -> (-58.1326, -70.2368) projected
  line L1317 (-58.1326, -70.2368) -> (-58.1326, -69.8368) projected
  line L1318 (-58.1326, -69.8368) -> (-57.3426, -69.8368) projected
  line L1319 (-57.3426, -69.8368) -> (-57.3426, -70.2368) projected
  line L1320 (-59.8826, -70.2368) -> (-60.6726, -70.2368) projected
  line L1321 (-60.6726, -70.2368) -> (-60.6726, -69.8368) projected
  line L1322 (-60.6726, -69.8368) -> (-59.8826, -69.8368) projected
  line L1323 (-59.8826, -69.8368) -> (-59.8826, -70.2368) projected
  line L1324 (-57.3426, -71.0368) -> (-58.1326, -71.0368) projected
  line L1325 (-58.1326, -71.0368) -> (-58.1326, -70.6368) projected
  line L1326 (-58.1326, -70.6368) -> (-57.3426, -70.6368) projected
  line L1327 (-57.3426, -70.6368) -> (-57.3426, -71.0368) projected
  line L1328 (-59.8826, -71.0368) -> (-60.6726, -71.0368) projected
  line L1329 (-60.6726, -71.0368) -> (-60.6726, -70.6368) projected
  line L1330 (-60.6726, -70.6368) -> (-59.8826, -70.6368) projected
  line L1331 (-59.8826, -70.6368) -> (-59.8826, -71.0368) projected
  line L1332 (-57.3426, -71.8368) -> (-58.1326, -71.8368) projected
  line L1333 (-58.1326, -71.8368) -> (-58.1326, -71.4368) projected
  line L1334 (-58.1326, -71.4368) -> (-57.3426, -71.4368) projected
  line L1335 (-57.3426, -71.4368) -> (-57.3426, -71.8368) projected
  line L1336 (-59.8826, -71.8368) -> (-60.6726, -71.8368) projected
  line L1337 (-60.6726, -71.8368) -> (-60.6726, -71.4368) projected
  line L1338 (-60.6726, -71.4368) -> (-59.8826, -71.4368) projected
  line L1339 (-59.8826, -71.4368) -> (-59.8826, -71.8368) projected
  line L1340 (-57.3426, -72.6368) -> (-58.1326, -72.6368) projected
  line L1341 (-58.1326, -72.6368) -> (-58.1326, -72.2368) projected
  line L1342 (-58.1326, -72.2368) -> (-57.3426, -72.2368) projected
  line L1343 (-57.3426, -72.2368) -> (-57.3426, -72.6368) projected
  line L1344 (-59.8826, -72.6368) -> (-60.6726, -72.6368) projected
  line L1345 (-60.6726, -72.6368) -> (-60.6726, -72.2368) projected
  line L1346 (-60.6726, -72.2368) -> (-59.8826, -72.2368) projected
  line L1347 (-59.8826, -72.2368) -> (-59.8826, -72.6368) projected
  line L1348 (-57.3426, -73.4368) -> (-58.1326, -73.4368) projected
  line L1349 (-58.1326, -73.4368) -> (-58.1326, -73.0368) projected
  line L1350 (-58.1326, -73.0368) -> (-57.3426, -73.0368) projected
  line L1351 (-57.3426, -73.0368) -> (-57.3426, -73.4368) projected
  line L1352 (-59.8826, -73.4368) -> (-60.6726, -73.4368) projected
  line L1353 (-60.6726, -73.4368) -> (-60.6726, -73.0368) projected
  line L1354 (-60.6726, -73.0368) -> (-59.8826, -73.0368) projected
  line L1355 (-59.8826, -73.0368) -> (-59.8826, -73.4368) projected
  line L1356 (-57.3426, -74.2368) -> (-58.1326, -74.2368) projected
  line L1357 (-58.1326, -74.2368) -> (-58.1326, -73.8368) projected
  line L1358 (-58.1326, -73.8368) -> (-57.3426, -73.8368) projected
  line L1359 (-57.3426, -73.8368) -> (-57.3426, -74.2368) projected
  line L1360 (-59.8826, -74.2368) -> (-60.6726, -74.2368) projected
  line L1361 (-60.6726, -74.2368) -> (-60.6726, -73.8368) projected
  line L1362 (-60.6726, -73.8368) -> (-59.8826, -73.8368) projected
  line L1363 (-59.8826, -73.8368) -> (-59.8826, -74.2368) projected
  line L1364 (-57.3426, -75.0368) -> (-58.1326, -75.0368) projected
  line L1365 (-58.1326, -75.0368) -> (-58.1326, -74.6368) projected
  line L1366 (-58.1326, -74.6368) -> (-57.3426, -74.6368) projected
  line L1367 (-57.3426, -74.6368) -> (-57.3426, -75.0368) projected
  line L1368 (-59.8826, -75.0368) -> (-60.6726, -75.0368) projected
  line L1369 (-60.6726, -75.0368) -> (-60.6726, -74.6368) projected
  line L1370 (-60.6726, -74.6368) -> (-59.8826, -74.6368) projected
  line L1371 (-59.8826, -74.6368) -> (-59.8826, -75.0368) projected
  line L1372 (-97.4501, -19.3368) -> (-95.8501, -19.3368) projected
  line L1373 (-95.8501, -19.3368) -> (-95.8501, -19.9868) projected
  line L1374 (-95.8501, -19.9868) -> (-97.4501, -19.9868) projected
  line L1375 (-97.4501, -19.9868) -> (-97.4501, -19.3368) projected
  line L1376 (-97.4501, -11.4368) -> (-95.8501, -11.4368) projected
  line L1377 (-95.8501, -11.4368) -> (-95.8501, -12.0868) projected
  line L1378 (-95.8501, -12.0868) -> (-97.4501, -12.0868) projected
  line L1379 (-97.4501, -12.0868) -> (-97.4501, -11.4368) projected
  line L1380 (-98.3151, -18.3118) -> (-97.5251, -18.3118) projected
  line L1381 (-97.5251, -18.3118) -> (-97.5251, -18.7118) projected
  line L1382 (-97.5251, -18.7118) -> (-98.3151, -18.7118) projected
  line L1383 (-98.3151, -18.7118) -> (-98.3151, -18.3118) projected
  line L1384 (-95.7751, -18.3118) -> (-94.9851, -18.3118) projected
  line L1385 (-94.9851, -18.3118) -> (-94.9851, -18.7118) projected
  line L1386 (-94.9851, -18.7118) -> (-95.7751, -18.7118) projected
  line L1387 (-95.7751, -18.7118) -> (-95.7751, -18.3118) projected
  line L1388 (-98.3151, -17.5118) -> (-97.5251, -17.5118) projected
  line L1389 (-97.5251, -17.5118) -> (-97.5251, -17.9118) projected
  line L1390 (-97.5251, -17.9118) -> (-98.3151, -17.9118) projected
  line L1391 (-98.3151, -17.9118) -> (-98.3151, -17.5118) projected
  line L1392 (-95.7751, -17.5118) -> (-94.9851, -17.5118) projected
  line L1393 (-94.9851, -17.5118) -> (-94.9851, -17.9118) projected
  line L1394 (-94.9851, -17.9118) -> (-95.7751, -17.9118) projected
  line L1395 (-95.7751, -17.9118) -> (-95.7751, -17.5118) projected
  line L1396 (-98.3151, -16.7118) -> (-97.5251, -16.7118) projected
  line L1397 (-97.5251, -16.7118) -> (-97.5251, -17.1118) projected
  line L1398 (-97.5251, -17.1118) -> (-98.3151, -17.1118) projected
  line L1399 (-98.3151, -17.1118) -> (-98.3151, -16.7118) projected
  line L1400 (-95.7751, -16.7118) -> (-94.9851, -16.7118) projected
  line L1401 (-94.9851, -16.7118) -> (-94.9851, -17.1118) projected
  line L1402 (-94.9851, -17.1118) -> (-95.7751, -17.1118) projected
  line L1403 (-95.7751, -17.1118) -> (-95.7751, -16.7118) projected
  line L1404 (-98.3151, -15.9118) -> (-97.5251, -15.9118) projected
  line L1405 (-97.5251, -15.9118) -> (-97.5251, -16.3118) projected
  line L1406 (-97.5251, -16.3118) -> (-98.3151, -16.3118) projected
  line L1407 (-98.3151, -16.3118) -> (-98.3151, -15.9118) projected
  line L1408 (-95.7751, -15.9118) -> (-94.9851, -15.9118) projected
  line L1409 (-94.9851, -15.9118) -> (-94.9851, -16.3118) projected
  line L1410 (-94.9851, -16.3118) -> (-95.7751, -16.3118) projected
  line L1411 (-95.7751, -16.3118) -> (-95.7751, -15.9118) projected
  line L1412 (-98.3151, -15.1118) -> (-97.5251, -15.1118) projected
  line L1413 (-97.5251, -15.1118) -> (-97.5251, -15.5118) projected
  line L1414 (-97.5251, -15.5118) -> (-98.3151, -15.5118) projected
  line L1415 (-98.3151, -15.5118) -> (-98.3151, -15.1118) projected
  line L1416 (-95.7751, -15.1118) -> (-94.9851, -15.1118) projected
  line L1417 (-94.9851, -15.1118) -> (-94.9851, -15.5118) projected
  line L1418 (-94.9851, -15.5118) -> (-95.7751, -15.5118) projected
  line L1419 (-95.7751, -15.5118) -> (-95.7751, -15.1118) projected
  line L1420 (-98.3151, -14.3118) -> (-97.5251, -14.3118) projected
  line L1421 (-97.5251, -14.3118) -> (-97.5251, -14.7118) projected
  line L1422 (-97.5251, -14.7118) -> (-98.3151, -14.7118) projected
  line L1423 (-98.3151, -14.7118) -> (-98.3151, -14.3118) projected
  line L1424 (-95.7751, -14.3118) -> (-94.9851, -14.3118) projected
  line L1425 (-94.9851, -14.3118) -> (-94.9851, -14.7118) projected
  line L1426 (-94.9851, -14.7118) -> (-95.7751, -14.7118) projected
  line L1427 (-95.7751, -14.7118) -> (-95.7751, -14.3118) projected
  line L1428 (-98.3151, -13.5118) -> (-97.5251, -13.5118) projected
  line L1429 (-97.5251, -13.5118) -> (-97.5251, -13.9118) projected
  line L1430 (-97.5251, -13.9118) -> (-98.3151, -13.9118) projected
  line L1431 (-98.3151, -13.9118) -> (-98.3151, -13.5118) projected
  line L1432 (-95.7751, -13.5118) -> (-94.9851, -13.5118) projected
  line L1433 (-94.9851, -13.5118) -> (-94.9851, -13.9118) projected
  line L1434 (-94.9851, -13.9118) -> (-95.7751, -13.9118) projected
  line L1435 (-95.7751, -13.9118) -> (-95.7751, -13.5118) projected
  line L1436 (-98.3151, -12.7118) -> (-97.5251, -12.7118) projected
  line L1437 (-97.5251, -12.7118) -> (-97.5251, -13.1118) projected
  line L1438 (-97.5251, -13.1118) -> (-98.3151, -13.1118) projected
  line L1439 (-98.3151, -13.1118) -> (-98.3151, -12.7118) projected
  line L1440 (-95.7751, -12.7118) -> (-94.9851, -12.7118) projected
  line L1441 (-94.9851, -12.7118) -> (-94.9851, -13.1118) projected
  line L1442 (-94.9851, -13.1118) -> (-95.7751, -13.1118) projected
  line L1443 (-95.7751, -13.1118) -> (-95.7751, -12.7118) projected
  line L1444 (-20.4076, -30.7618) -> (-22.0076, -30.7618) projected
  line L1445 (-22.0076, -30.7618) -> (-22.0076, -30.1118) projected
  line L1446 (-22.0076, -30.1118) -> (-20.4076, -30.1118) projected
  line L1447 (-20.4076, -30.1118) -> (-20.4076, -30.7618) projected
  line L1448 (-20.4076, -38.6618) -> (-22.0076, -38.6618) projected
  line L1449 (-22.0076, -38.6618) -> (-22.0076, -38.0118) projected
  line L1450 (-22.0076, -38.0118) -> (-20.4076, -38.0118) projected
  line L1451 (-20.4076, -38.0118) -> (-20.4076, -38.6618) projected
  line L1452 (-19.5426, -31.7868) -> (-20.3326, -31.7868) projected
  line L1453 (-20.3326, -31.7868) -> (-20.3326, -31.3868) projected
  line L1454 (-20.3326, -31.3868) -> (-19.5426, -31.3868) projected
  line L1455 (-19.5426, -31.3868) -> (-19.5426, -31.7868) projected
  line L1456 (-22.0826, -31.7868) -> (-22.8726, -31.7868) projected
  line L1457 (-22.8726, -31.7868) -> (-22.8726, -31.3868) projected
  line L1458 (-22.8726, -31.3868) -> (-22.0826, -31.3868) projected
  line L1459 (-22.0826, -31.3868) -> (-22.0826, -31.7868) projected
  line L1460 (-19.5426, -32.5868) -> (-20.3326, -32.5868) projected
  line L1461 (-20.3326, -32.5868) -> (-20.3326, -32.1868) projected
  line L1462 (-20.3326, -32.1868) -> (-19.5426, -32.1868) projected
  line L1463 (-19.5426, -32.1868) -> (-19.5426, -32.5868) projected
  line L1464 (-22.0826, -32.5868) -> (-22.8726, -32.5868) projected
  line L1465 (-22.8726, -32.5868) -> (-22.8726, -32.1868) projected
  line L1466 (-22.8726, -32.1868) -> (-22.0826, -32.1868) projected
  line L1467 (-22.0826, -32.1868) -> (-22.0826, -32.5868) projected
  line L1468 (-19.5426, -33.3868) -> (-20.3326, -33.3868) projected
  line L1469 (-20.3326, -33.3868) -> (-20.3326, -32.9868) projected
  line L1470 (-20.3326, -32.9868) -> (-19.5426, -32.9868) projected
  line L1471 (-19.5426, -32.9868) -> (-19.5426, -33.3868) projected
  line L1472 (-22.0826, -33.3868) -> (-22.8726, -33.3868) projected
  line L1473 (-22.8726, -33.3868) -> (-22.8726, -32.9868) projected
  line L1474 (-22.8726, -32.9868) -> (-22.0826, -32.9868) projected
  line L1475 (-22.0826, -32.9868) -> (-22.0826, -33.3868) projected
  line L1476 (-19.5426, -34.1868) -> (-20.3326, -34.1868) projected
  line L1477 (-20.3326, -34.1868) -> (-20.3326, -33.7868) projected
  line L1478 (-20.3326, -33.7868) -> (-19.5426, -33.7868) projected
  line L1479 (-19.5426, -33.7868) -> (-19.5426, -34.1868) projected
  line L1480 (-22.0826, -34.1868) -> (-22.8726, -34.1868) projected
  line L1481 (-22.8726, -34.1868) -> (-22.8726, -33.7868) projected
  line L1482 (-22.8726, -33.7868) -> (-22.0826, -33.7868) projected
  line L1483 (-22.0826, -33.7868) -> (-22.0826, -34.1868) projected
  line L1484 (-19.5426, -34.9868) -> (-20.3326, -34.9868) projected
  line L1485 (-20.3326, -34.9868) -> (-20.3326, -34.5868) projected
  line L1486 (-20.3326, -34.5868) -> (-19.5426, -34.5868) projected
  line L1487 (-19.5426, -34.5868) -> (-19.5426, -34.9868) projected
  line L1488 (-22.0826, -34.9868) -> (-22.8726, -34.9868) projected
  line L1489 (-22.8726, -34.9868) -> (-22.8726, -34.5868) projected
  line L1490 (-22.8726, -34.5868) -> (-22.0826, -34.5868) projected
  line L1491 (-22.0826, -34.5868) -> (-22.0826, -34.9868) projected
  line L1492 (-19.5426, -35.7868) -> (-20.3326, -35.7868) projected
  line L1493 (-20.3326, -35.7868) -> (-20.3326, -35.3868) projected
  line L1494 (-20.3326, -35.3868) -> (-19.5426, -35.3868) projected
  line L1495 (-19.5426, -35.3868) -> (-19.5426, -35.7868) projected
  line L1496 (-22.0826, -35.7868) -> (-22.8726, -35.7868) projected
  line L1497 (-22.8726, -35.7868) -> (-22.8726, -35.3868) projected
  line L1498 (-22.8726, -35.3868) -> (-22.0826, -35.3868) projected
  line L1499 (-22.0826, -35.3868) -> (-22.0826, -35.7868) projected
  line L1500 (-19.5426, -36.5868) -> (-20.3326, -36.5868) projected
  line L1501 (-20.3326, -36.5868) -> (-20.3326, -36.1868) projected
  line L1502 (-20.3326, -36.1868) -> (-19.5426, -36.1868) projected
  line L1503 (-19.5426, -36.1868) -> (-19.5426, -36.5868) projected
  line L1504 (-22.0826, -36.5868) -> (-22.8726, -36.5868) projected
  line L1505 (-22.8726, -36.5868) -> (-22.8726, -36.1868) projected
  line L1506 (-22.8726, -36.1868) -> (-22.0826, -36.1868) projected
  line L1507 (-22.0826, -36.1868) -> (-22.0826, -36.5868) projected
  line L1508 (-19.5426, -37.3868) -> (-20.3326, -37.3868) projected
  line L1509 (-20.3326, -37.3868) -> (-20.3326, -36.9868) projected
  line L1510 (-20.3326, -36.9868) -> (-19.5426, -36.9868) projected
  line L1511 (-19.5426, -36.9868) -> (-19.5426, -37.3868) projected
  line L1512 (-22.0826, -37.3868) -> (-22.8726, -37.3868) projected
  line L1513 (-22.8726, -37.3868) -> (-22.8726, -36.9868) projected
  line L1514 (-22.8726, -36.9868) -> (-22.0826, -36.9868) projected
  line L1515 (-22.0826, -36.9868) -> (-22.0826, -37.3868) projected
  line L1516 (-114.7201, -30.6868) -> (-116.3201, -30.6868) projected
  line L1517 (-116.3201, -30.6868) -> (-116.3201, -30.0368) projected
  line L1518 (-116.3201, -30.0368) -> (-114.7201, -30.0368) projected
  line L1519 (-114.7201, -30.0368) -> (-114.7201, -30.6868) projected
  line L1520 (-114.7201, -38.5868) -> (-116.3201, -38.5868) projected
  line L1521 (-116.3201, -38.5868) -> (-116.3201, -37.9368) projected
  line L1522 (-116.3201, -37.9368) -> (-114.7201, -37.9368) projected
  line L1523 (-114.7201, -37.9368) -> (-114.7201, -38.5868) projected
  line L1524 (-113.8551, -31.7118) -> (-114.6451, -31.7118) projected
  line L1525 (-114.6451, -31.7118) -> (-114.6451, -31.3118) projected
  line L1526 (-114.6451, -31.3118) -> (-113.8551, -31.3118) projected
  line L1527 (-113.8551, -31.3118) -> (-113.8551, -31.7118) projected
  line L1528 (-116.3951, -31.7118) -> (-117.1851, -31.7118) projected
  line L1529 (-117.1851, -31.7118) -> (-117.1851, -31.3118) projected
  line L1530 (-117.1851, -31.3118) -> (-116.3951, -31.3118) projected
  line L1531 (-116.3951, -31.3118) -> (-116.3951, -31.7118) projected
  line L1532 (-113.8551, -32.5118) -> (-114.6451, -32.5118) projected
  line L1533 (-114.6451, -32.5118) -> (-114.6451, -32.1118) projected
  line L1534 (-114.6451, -32.1118) -> (-113.8551, -32.1118) projected
  line L1535 (-113.8551, -32.1118) -> (-113.8551, -32.5118) projected
  line L1536 (-116.3951, -32.5118) -> (-117.1851, -32.5118) projected
  line L1537 (-117.1851, -32.5118) -> (-117.1851, -32.1118) projected
  line L1538 (-117.1851, -32.1118) -> (-116.3951, -32.1118) projected
  line L1539 (-116.3951, -32.1118) -> (-116.3951, -32.5118) projected
  line L1540 (-113.8551, -33.3118) -> (-114.6451, -33.3118) projected
  line L1541 (-114.6451, -33.3118) -> (-114.6451, -32.9118) projected
  line L1542 (-114.6451, -32.9118) -> (-113.8551, -32.9118) projected
  line L1543 (-113.8551, -32.9118) -> (-113.8551, -33.3118) projected
  line L1544 (-116.3951, -33.3118) -> (-117.1851, -33.3118) projected
  line L1545 (-117.1851, -33.3118) -> (-117.1851, -32.9118) projected
  line L1546 (-117.1851, -32.9118) -> (-116.3951, -32.9118) projected
  line L1547 (-116.3951, -32.9118) -> (-116.3951, -33.3118) projected
  line L1548 (-113.8551, -34.1118) -> (-114.6451, -34.1118) projected
  line L1549 (-114.6451, -34.1118) -> (-114.6451, -33.7118) projected
  line L1550 (-114.6451, -33.7118) -> (-113.8551, -33.7118) projected
  line L1551 (-113.8551, -33.7118) -> (-113.8551, -34.1118) projected
  line L1552 (-116.3951, -34.1118) -> (-117.1851, -34.1118) projected
  line L1553 (-117.1851, -34.1118) -> (-117.1851, -33.7118) projected
  line L1554 (-117.1851, -33.7118) -> (-116.3951, -33.7118) projected
  line L1555 (-116.3951, -33.7118) -> (-116.3951, -34.1118) projected
  line L1556 (-113.8551, -34.9118) -> (-114.6451, -34.9118) projected
  line L1557 (-114.6451, -34.9118) -> (-114.6451, -34.5118) projected
  line L1558 (-114.6451, -34.5118) -> (-113.8551, -34.5118) projected
  line L1559 (-113.8551, -34.5118) -> (-113.8551, -34.9118) projected
  line L1560 (-116.3951, -34.9118) -> (-117.1851, -34.9118) projected
  line L1561 (-117.1851, -34.9118) -> (-117.1851, -34.5118) projected
  line L1562 (-117.1851, -34.5118) -> (-116.3951, -34.5118) projected
  line L1563 (-116.3951, -34.5118) -> (-116.3951, -34.9118) projected
  line L1564 (-113.8551, -35.7118) -> (-114.6451, -35.7118) projected
  line L1565 (-114.6451, -35.7118) -> (-114.6451, -35.3118) projected
  line L1566 (-114.6451, -35.3118) -> (-113.8551, -35.3118) projected
  line L1567 (-113.8551, -35.3118) -> (-113.8551, -35.7118) projected
  line L1568 (-116.3951, -35.7118) -> (-117.1851, -35.7118) projected
  line L1569 (-117.1851, -35.7118) -> (-117.1851, -35.3118) projected
  line L1570 (-117.1851, -35.3118) -> (-116.3951, -35.3118) projected
  line L1571 (-116.3951, -35.3118) -> (-116.3951, -35.7118) projected
  line L1572 (-113.8551, -36.5118) -> (-114.6451, -36.5118) projected
  line L1573 (-114.6451, -36.5118) -> (-114.6451, -36.1118) projected
  line L1574 (-114.6451, -36.1118) -> (-113.8551, -36.1118) projected
  line L1575 (-113.8551, -36.1118) -> (-113.8551, -36.5118) projected
  line L1576 (-116.3951, -36.5118) -> (-117.1851, -36.5118) projected
  line L1577 (-117.1851, -36.5118) -> (-117.1851, -36.1118) projected
  line L1578 (-117.1851, -36.1118) -> (-116.3951, -36.1118) projected
  line L1579 (-116.3951, -36.1118) -> (-116.3951, -36.5118) projected
  line L1580 (-113.8551, -37.3118) -> (-114.6451, -37.3118) projected
  line L1581 (-114.6451, -37.3118) -> (-114.6451, -36.9118) projected
  line L1582 (-114.6451, -36.9118) -> (-113.8551, -36.9118) projected
  line L1583 (-113.8551, -36.9118) -> (-113.8551, -37.3118) projected
  line L1584 (-116.3951, -37.3118) -> (-117.1851, -37.3118) projected
  line L1585 (-117.1851, -37.3118) -> (-117.1851, -36.9118) projected
  line L1586 (-117.1851, -36.9118) -> (-116.3951, -36.9118) projected
  line L1587 (-116.3951, -36.9118) -> (-116.3951, -37.3118) projected
  line L1588 (-20.3326, -68.5368) -> (-21.9326, -68.5368) projected
  line L1589 (-21.9326, -68.5368) -> (-21.9326, -67.8868) projected
  line L1590 (-21.9326, -67.8868) -> (-20.3326, -67.8868) projected
  line L1591 (-20.3326, -67.8868) -> (-20.3326, -68.5368) projected
  line L1592 (-20.3326, -76.4368) -> (-21.9326, -76.4368) projected
  line L1593 (-21.9326, -76.4368) -> (-21.9326, -75.7868) projected
  line L1594 (-21.9326, -75.7868) -> (-20.3326, -75.7868) projected
  line L1595 (-20.3326, -75.7868) -> (-20.3326, -76.4368) projected
  line L1596 (-19.4676, -69.5618) -> (-20.2576, -69.5618) projected
  line L1597 (-20.2576, -69.5618) -> (-20.2576, -69.1618) projected
  line L1598 (-20.2576, -69.1618) -> (-19.4676, -69.1618) projected
  line L1599 (-19.4676, -69.1618) -> (-19.4676, -69.5618) projected
  line L1600 (-22.0076, -69.5618) -> (-22.7976, -69.5618) projected
  line L1601 (-22.7976, -69.5618) -> (-22.7976, -69.1618) projected
  line L1602 (-22.7976, -69.1618) -> (-22.0076, -69.1618) projected
  line L1603 (-22.0076, -69.1618) -> (-22.0076, -69.5618) projected
  line L1604 (-19.4676, -70.3618) -> (-20.2576, -70.3618) projected
  line L1605 (-20.2576, -70.3618) -> (-20.2576, -69.9618) projected
  line L1606 (-20.2576, -69.9618) -> (-19.4676, -69.9618) projected
  line L1607 (-19.4676, -69.9618) -> (-19.4676, -70.3618) projected
  line L1608 (-22.0076, -70.3618) -> (-22.7976, -70.3618) projected
  line L1609 (-22.7976, -70.3618) -> (-22.7976, -69.9618) projected
  line L1610 (-22.7976, -69.9618) -> (-22.0076, -69.9618) projected
  line L1611 (-22.0076, -69.9618) -> (-22.0076, -70.3618) projected
  line L1612 (-19.4676, -71.1618) -> (-20.2576, -71.1618) projected
  line L1613 (-20.2576, -71.1618) -> (-20.2576, -70.7618) projected
  line L1614 (-20.2576, -70.7618) -> (-19.4676, -70.7618) projected
  line L1615 (-19.4676, -70.7618) -> (-19.4676, -71.1618) projected
  line L1616 (-22.0076, -71.1618) -> (-22.7976, -71.1618) projected
  line L1617 (-22.7976, -71.1618) -> (-22.7976, -70.7618) projected
  line L1618 (-22.7976, -70.7618) -> (-22.0076, -70.7618) projected
  line L1619 (-22.0076, -70.7618) -> (-22.0076, -71.1618) projected
  line L1620 (-19.4676, -71.9618) -> (-20.2576, -71.9618) projected
  line L1621 (-20.2576, -71.9618) -> (-20.2576, -71.5618) projected
  line L1622 (-20.2576, -71.5618) -> (-19.4676, -71.5618) projected
  line L1623 (-19.4676, -71.5618) -> (-19.4676, -71.9618) projected
  line L1624 (-22.0076, -71.9618) -> (-22.7976, -71.9618) projected
  line L1625 (-22.7976, -71.9618) -> (-22.7976, -71.5618) projected
  line L1626 (-22.7976, -71.5618) -> (-22.0076, -71.5618) projected
  line L1627 (-22.0076, -71.5618) -> (-22.0076, -71.9618) projected
  line L1628 (-19.4676, -72.7618) -> (-20.2576, -72.7618) projected
  line L1629 (-20.2576, -72.7618) -> (-20.2576, -72.3618) projected
  line L1630 (-20.2576, -72.3618) -> (-19.4676, -72.3618) projected
  line L1631 (-19.4676, -72.3618) -> (-19.4676, -72.7618) projected
  line L1632 (-22.0076, -72.7618) -> (-22.7976, -72.7618) projected
  line L1633 (-22.7976, -72.7618) -> (-22.7976, -72.3618) projected
  line L1634 (-22.7976, -72.3618) -> (-22.0076, -72.3618) projected
  line L1635 (-22.0076, -72.3618) -> (-22.0076, -72.7618) projected
  line L1636 (-19.4676, -73.5618) -> (-20.2576, -73.5618) projected
  line L1637 (-20.2576, -73.5618) -> (-20.2576, -73.1618) projected
  line L1638 (-20.2576, -73.1618) -> (-19.4676, -73.1618) projected
  line L1639 (-19.4676, -73.1618) -> (-19.4676, -73.5618) projected
  line L1640 (-22.0076, -73.5618) -> (-22.7976, -73.5618) projected
  line L1641 (-22.7976, -73.5618) -> (-22.7976, -73.1618) projected
  line L1642 (-22.7976, -73.1618) -> (-22.0076, -73.1618) projected
  line L1643 (-22.0076, -73.1618) -> (-22.0076, -73.5618) projected
  line L1644 (-19.4676, -74.3618) -> (-20.2576, -74.3618) projected
  line L1645 (-20.2576, -74.3618) -> (-20.2576, -73.9618) projected
  line L1646 (-20.2576, -73.9618) -> (-19.4676, -73.9618) projected
  line L1647 (-19.4676, -73.9618) -> (-19.4676, -74.3618) projected
  line L1648 (-22.0076, -74.3618) -> (-22.7976, -74.3618) projected
  line L1649 (-22.7976, -74.3618) -> (-22.7976, -73.9618) projected
  line L1650 (-22.7976, -73.9618) -> (-22.0076, -73.9618) projected
  line L1651 (-22.0076, -73.9618) -> (-22.0076, -74.3618) projected
  line L1652 (-19.4676, -75.1618) -> (-20.2576, -75.1618) projected
  line L1653 (-20.2576, -75.1618) -> (-20.2576, -74.7618) projected
  line L1654 (-20.2576, -74.7618) -> (-19.4676, -74.7618) projected
  line L1655 (-19.4676, -74.7618) -> (-19.4676, -75.1618) projected
  line L1656 (-22.0076, -75.1618) -> (-22.7976, -75.1618) projected
  line L1657 (-22.7976, -75.1618) -> (-22.7976, -74.7618) projected
  line L1658 (-22.7976, -74.7618) -> (-22.0076, -74.7618) projected
  line L1659 (-22.0076, -74.7618) -> (-22.0076, -75.1618) projected
  line L1660 (-77.1576, -30.6368) -> (-78.7576, -30.6368) projected
  line L1661 (-78.7576, -30.6368) -> (-78.7576, -29.9868) projected
  line L1662 (-78.7576, -29.9868) -> (-77.1576, -29.9868) projected
  line L1663 (-77.1576, -29.9868) -> (-77.1576, -30.6368) projected
  line L1664 (-77.1576, -38.5368) -> (-78.7576, -38.5368) projected
  line L1665 (-78.7576, -38.5368) -> (-78.7576, -37.8868) projected
  line L1666 (-78.7576, -37.8868) -> (-77.1576, -37.8868) projected
  line L1667 (-77.1576, -37.8868) -> (-77.1576, -38.5368) projected
  line L1668 (-76.2926, -31.6618) -> (-77.0826, -31.6618) projected
  line L1669 (-77.0826, -31.6618) -> (-77.0826, -31.2618) projected
  line L1670 (-77.0826, -31.2618) -> (-76.2926, -31.2618) projected
  line L1671 (-76.2926, -31.2618) -> (-76.2926, -31.6618) projected
  line L1672 (-78.8326, -31.6618) -> (-79.6226, -31.6618) projected
  line L1673 (-79.6226, -31.6618) -> (-79.6226, -31.2618) projected
  line L1674 (-79.6226, -31.2618) -> (-78.8326, -31.2618) projected
  line L1675 (-78.8326, -31.2618) -> (-78.8326, -31.6618) projected
  line L1676 (-76.2926, -32.4618) -> (-77.0826, -32.4618) projected
  line L1677 (-77.0826, -32.4618) -> (-77.0826, -32.0618) projected
  line L1678 (-77.0826, -32.0618) -> (-76.2926, -32.0618) projected
  line L1679 (-76.2926, -32.0618) -> (-76.2926, -32.4618) projected
  line L1680 (-78.8326, -32.4618) -> (-79.6226, -32.4618) projected
  line L1681 (-79.6226, -32.4618) -> (-79.6226, -32.0618) projected
  line L1682 (-79.6226, -32.0618) -> (-78.8326, -32.0618) projected
  line L1683 (-78.8326, -32.0618) -> (-78.8326, -32.4618) projected
  line L1684 (-76.2926, -33.2618) -> (-77.0826, -33.2618) projected
  line L1685 (-77.0826, -33.2618) -> (-77.0826, -32.8618) projected
  line L1686 (-77.0826, -32.8618) -> (-76.2926, -32.8618) projected
  line L1687 (-76.2926, -32.8618) -> (-76.2926, -33.2618) projected
  line L1688 (-78.8326, -33.2618) -> (-79.6226, -33.2618) projected
  line L1689 (-79.6226, -33.2618) -> (-79.6226, -32.8618) projected
  line L1690 (-79.6226, -32.8618) -> (-78.8326, -32.8618) projected
  line L1691 (-78.8326, -32.8618) -> (-78.8326, -33.2618) projected
  line L1692 (-76.2926, -34.0618) -> (-77.0826, -34.0618) projected
  line L1693 (-77.0826, -34.0618) -> (-77.0826, -33.6618) projected
  line L1694 (-77.0826, -33.6618) -> (-76.2926, -33.6618) projected
  line L1695 (-76.2926, -33.6618) -> (-76.2926, -34.0618) projected
  line L1696 (-78.8326, -34.0618) -> (-79.6226, -34.0618) projected
  line L1697 (-79.6226, -34.0618) -> (-79.6226, -33.6618) projected
  line L1698 (-79.6226, -33.6618) -> (-78.8326, -33.6618) projected
  line L1699 (-78.8326, -33.6618) -> (-78.8326, -34.0618) projected
  line L1700 (-76.2926, -34.8618) -> (-77.0826, -34.8618) projected
  line L1701 (-77.0826, -34.8618) -> (-77.0826, -34.4618) projected
  line L1702 (-77.0826, -34.4618) -> (-76.2926, -34.4618) projected
  line L1703 (-76.2926, -34.4618) -> (-76.2926, -34.8618) projected
  line L1704 (-78.8326, -34.8618) -> (-79.6226, -34.8618) projected
  line L1705 (-79.6226, -34.8618) -> (-79.6226, -34.4618) projected
  line L1706 (-79.6226, -34.4618) -> (-78.8326, -34.4618) projected
  line L1707 (-78.8326, -34.4618) -> (-78.8326, -34.8618) projected
  line L1708 (-76.2926, -35.6618) -> (-77.0826, -35.6618) projected
  line L1709 (-77.0826, -35.6618) -> (-77.0826, -35.2618) projected
  line L1710 (-77.0826, -35.2618) -> (-76.2926, -35.2618) projected
  line L1711 (-76.2926, -35.2618) -> (-76.2926, -35.6618) projected
  line L1712 (-78.8326, -35.6618) -> (-79.6226, -35.6618) projected
  line L1713 (-79.6226, -35.6618) -> (-79.6226, -35.2618) projected
  line L1714 (-79.6226, -35.2618) -> (-78.8326, -35.2618) projected
  line L1715 (-78.8326, -35.2618) -> (-78.8326, -35.6618) projected
  line L1716 (-76.2926, -36.4618) -> (-77.0826, -36.4618) projected
  line L1717 (-77.0826, -36.4618) -> (-77.0826, -36.0618) projected
  line L1718 (-77.0826, -36.0618) -> (-76.2926, -36.0618) projected
  line L1719 (-76.2926, -36.0618) -> (-76.2926, -36.4618) projected
  line L1720 (-78.8326, -36.4618) -> (-79.6226, -36.4618) projected
  line L1721 (-79.6226, -36.4618) -> (-79.6226, -36.0618) projected
  line L1722 (-79.6226, -36.0618) -> (-78.8326, -36.0618) projected
  line L1723 (-78.8326, -36.0618) -> (-78.8326, -36.4618) projected
  line L1724 (-76.2926, -37.2618) -> (-77.0826, -37.2618) projected
  line L1725 (-77.0826, -37.2618) -> (-77.0826, -36.8618) projected
  line L1726 (-77.0826, -36.8618) -> (-76.2926, -36.8618) projected
  line L1727 (-76.2926, -36.8618) -> (-76.2926, -37.2618) projected